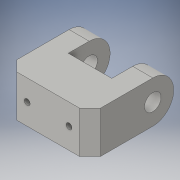
# Autodesk Inventor part: band_hinge
Saved by Autodesk Inventor 2016 (Build 200138000, 138)
## iProperties
Created: 2016-02-24
Part Number: band_hinge
Material: Generic
Document SubType Name: Modeling
Designer: Matt Ruffner
Density: 1 g/cm^3
Appearance: Default
Author: Matt Ruffner
Autodesk Inventor part; units mm, degrees
ref_plane "YZ Plane" through (0, 0, 0) normal (1, 0, 0) x (0, 1, 0)
ref_plane "XZ Plane" through (0, 0, 0) normal (0, 1, 0) x (-1, 0, 0)
ref_plane "XY Plane" through (0, 0, 0) normal (0, 0, 1) x (1, 0, 0)
sketch "Sketch1" plane through (0, 0, 0) normal (1, 0, 0) x (0, 1, 0)
  line L0 (4.6679, 5.5772) -> (-8.0321, 5.5772)
  line L1 (-8.0321, 5.5772) -> (-8.0321, -13.4728)
  line L2 (-1.6821, -19.8228) -> (-1.6821, -19.8228)
  line L3 (4.6679, -13.4728) -> (4.6679, 5.5772)
  circle A0 centre (-1.6821, -13.4728) radius 2.5083
  arc A1 (-1.6821, -19.8228) -> (4.6679, -13.4728) centre (-1.6821, -13.4728) ccw
  arc A2 (-8.0321, -13.4728) -> (-1.6821, -19.8228) centre (-1.6821, -13.4728) ccw
  point P0 (0, 0)
  point P1 (-8.0321, -19.8228)
  point P2 (4.6679, -19.8228)
  dimension "d0" = 12.7
  dimension "d1" = 25.4
  dimension "d2" = 5.0165
  dimension "d3" = 6.35
  dimension "d4" = 6.35
  constraints: 8 end point, 4 point on circle, 4 point on line, 4 tangent, 3 centre point, 2 parallel, 1 concentric, 1 horizontal, 1 perpendicular
  measures "d0" distance of point (4.668, -19.823) point (-8.032, -19.823)
  measures "d1" distance of point (-8.032, -19.823) L0.end
  measures "d2" diameter of A0
  measures "d3" distance from line of L2 A0.centre
  measures "d4" radius of A1
extrude "Extrusion1" add sketch "Sketch1" against normal blind 25.4
sketch "Sketch2" plane through (0, -8.0321, 5.5772) normal (0, 0, 1) x (1, 0, 0)
  line L0 (0, 0) -> (-25.4, 0) projected
  line L1 (0, 12.7) -> (0, 0) projected
  circle A0 centre (-6.35, 6.35) radius 0.889
  circle A1 centre (-19.05, 6.35) radius 0.889
  line L2 (-25.4, 0) -> (-25.4, 12.7) projected
  point P0 (0, 8.0321)
  point P1 (-12.7, 6.35)
  dimension "d7" = 6.35
  dimension "d8" = 12.7
  dimension "d9" = 1.778
  dimension "d10" = 6.35
  dimension "d11" = 1.778
  dimension "d12" = 6.35
  constraints: 2 centre point
  measures "d7" distance from line of L0 point (-12.7, 6.35)
  measures "d8" distance from line of L1 point (-12.7, 6.35)
  measures "d9" diameter of A0
  measures "d10" distance from line of L1 A0.centre
  measures "d11" diameter of A1
  measures "d12" distance from line of L2 A1.centre
extrude "Extrusion2" cut sketch "Sketch2" against normal blind 11.43
chamfer "Chamfer1" distance 3.175 angle 45 2 edges at (0, -1.6821, 5.5772) (-25.4, -1.6821, 5.5772)
sketch "Sketch3" plane through (-25.4, 4.6679, -13.4728) normal (0, 1, 0) x (1, 0, 0)
  line L0 (25.4, 6.35) -> (0, 6.35) projected
  line L1 (6.096, 6.35) -> (19.304, 6.35)
  line L2 (19.304, 6.35) -> (19.304, -6.35)
  line L3 (19.304, -6.35) -> (6.096, -6.35)
  line L4 (6.096, -6.35) -> (6.096, 6.35)
  line L5 (25.4, 0) -> (25.4, 6.35) projected
  line L6 (0, 6.35) -> (0, 0) projected
  point P0 (25.4, -13.4728)
  dimension "d18" = 12.7
  dimension "d19" = 6.096
  dimension "d20" = 6.096
  constraints: 8 end point, 2 parallel, 1 horizontal, 1 perpendicular, 1 point on line
  measures "d18" distance between parallel lines of L0 L3
  measures "d19" distance between parallel lines of L5 L2
  measures "d20" distance between parallel lines of L6 L4
extrude "Extrusion3" cut sketch "Sketch3" against normal blind 12.7
body "Solid1"
